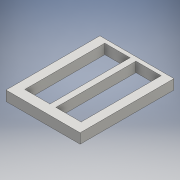
# Autodesk Inventor part: Fenetre-Bords
Saved by Autodesk Inventor 2016 SP1 (Build 200210100, 210)
## iProperties
Created: 2016-10-04
Part Number: Fenetre-Bords
Material: Plastique ABS
Document SubType Name: Modeling
Designer: dimercur
Density: 1.06 g/cm^3
Appearance: Lisse - Blanc
Mass: 604200 g
Surface Area: 70600 cm^2
Volume: 570000 cm^3
Author: dimercur
Autodesk Inventor part; units mm, degrees
ref_plane "YZ Plane" through (0, 0, 0) normal (1, 0, 0) x (0, 1, 0)
ref_plane "XZ Plane" through (0, 0, 0) normal (0, 1, 0) x (-1, 0, 0)
ref_plane "XY Plane" through (0, 0, 0) normal (0, 0, 1) x (1, 0, 0)
sketch "Esquisse1" plane through (0, 0, 0) normal (0, 0, 1) x (1, 0, 0)
  line L0 (-745.614, 899.1228) -> (754.386, 899.1228)
  line L1 (754.386, 899.1228) -> (754.386, -1000.8772)
  line L2 (754.386, -1000.8772) -> (-745.614, -1000.8772)
  line L3 (-745.614, -1000.8772) -> (-745.614, 899.1228)
  point P0 (0, 0)
  dimension "d0" = 1500
  dimension "d1" = 1900
  constraints: 8 end point, 2 parallel, 1 horizontal, 1 perpendicular
  measures "d0" distance of L0.start L0.end
  measures "d1" distance of L2.end L0.start
extrude "Extrusion1" add sketch "Esquisse1" along normal blind 200
sketch "Esquisse2" plane through (0, 0, 200) normal (0, 0, 1) x (1, 0, 0)
  line L0 (-565.614, 819.1228) -> (-55.614, 819.1228)
  line L1 (-55.614, 819.1228) -> (-55.614, -800.8772)
  line L2 (-55.614, -800.8772) -> (-565.614, -800.8772)
  line L3 (-565.614, -800.8772) -> (-565.614, 819.1228)
  line L4 (64.386, 819.1228) -> (574.386, 819.1228)
  line L5 (574.386, 819.1228) -> (574.386, -800.8772)
  line L6 (574.386, -800.8772) -> (64.386, -800.8772)
  line L7 (64.386, -800.8772) -> (64.386, 819.1228)
  line L8 (-745.614, 899.1228) -> (-745.614, -1000.8772) projected
  line L9 (754.386, -1000.8772) -> (754.386, 899.1228) projected
  line L10 (-745.614, -1000.8772) -> (754.386, -1000.8772) projected
  point P0 (0, 0)
  dimension "d4" = 510
  dimension "d5" = 510
  dimension "d6" = 1620
  dimension "d7" = 1620
  dimension "d8" = 180
  dimension "d9" = 180
  dimension "d10" = 200
  constraints: 16 end point, 4 parallel, 2 horizontal, 2 perpendicular, 1 point on line
  measures "d4" distance of L0.start L0.end
  measures "d5" distance of L4.start L4.end
  measures "d6" distance of L2.end L0.start
  measures "d7" distance of L4.end L5.end
  measures "d8" distance between parallel lines of L8 L3
  measures "d9" distance between parallel lines of L9 L5
  measures "d10" distance between parallel lines of L10 L2
extrude "Extrusion2" cut sketch "Esquisse2" against normal blind 200
